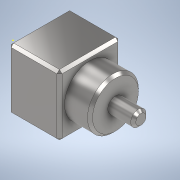
# Autodesk Inventor part: motor(1 shaft)
Saved by Autodesk Inventor 2021 (Build 250183000, 183)
## iProperties
Created: 2021-07-03
Part Number: motor(1 shaft)
Material: Steel, Alloy
Document SubType Name: Modeling
Designer: Prerana
Density: 7.73 g/cm^3
Appearance: Semi-Polished
Author: Prerana
Autodesk Inventor part; units mm, degrees
ref_plane "YZ Plane" through (0, 0, 0) normal (1, 0, 0) x (0, 1, 0)
ref_plane "XZ Plane" through (0, 0, 0) normal (0, 1, 0) x (-1, 0, 0)
ref_plane "XY Plane" through (0, 0, 0) normal (0, 0, 1) x (1, 0, 0)
sketch "Sketch1" plane through (0, 0, 0) normal (0, 1, 0) x (-1, 0, 0)
  point P0 (0, 0)
sketch "Sketch2" plane through (0, 0, 0) normal (1, 0, 0) x (0, 1, 0)
  line L0 (1.9877, 1.8129) -> (-22.0123, 1.8129)
  line L1 (-22.0123, 1.8129) -> (-22.0123, -22.1871)
  line L2 (-22.0123, -22.1871) -> (1.9877, -22.1871)
  line L3 (1.9877, -22.1871) -> (1.9877, 1.8129)
  point P0 (0, 0)
  constraints: 8 end point, 2 parallel, 1 horizontal, 1 perpendicular
extrude "Extrusion1" add sketch "Sketch2" along normal blind 20
sketch "Sketch3" plane through (20, 0, 0) normal (1, 0, 0) x (0, 0, -1)
  circle A0 centre (10.1871, -10.0123) radius 10
  line L0 (22.1871, 1.9877) -> (-1.8129, 1.9877) projected
  line L1 (-1.8129, 1.9877) -> (-1.8129, -22.0123) projected
  point P0 (0, 0)
  constraints: 1 centre point
extrude "Extrusion2" add sketch "Sketch3" along normal blind 10
sketch "Sketch4" plane through (30, -10.0123, -10.1871) normal (1, 0, 0) x (0, 0, -1)
  circle A0 centre (0, 0) radius 3
  point P0 (-10.1871, 10.0123)
  constraints: 1 centre point
extrude "Extrusion3" add sketch "Sketch4" along normal blind 10
chamfer "Chamfer1" distance 1 angle 45 13 edges at (0, 1.9877, -10.1871) (10, 1.9877, -22.1871) (20, 1.9877, -10.1871) (10, 1.9877, 1.8129) (20, -10.0123, 1.8129) (20, -10.0123, -22.1871) (30, -10.0123, -0.1871) (40, -10.0123, -7.1871) (0, -10.0123, 1.8129) (10, -22.0123, 1.8129) (20, -22.0123, -10.1871) (0, -10.0123, -22.1871) (0, -22.0123, -10.1871)
sketch "Sketch5" plane through (1, 1.9877, 0.8129) normal (0, 1, 0) x (1, 0, 0)
  point P0 (-1, 0.8129)
body "Solid1"
